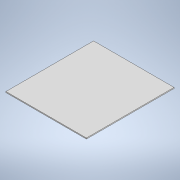
# Autodesk Inventor part: casing lidN
Saved by Autodesk Inventor 2022 (Build 260153000, 153)
## iProperties
Created: 2023-02-15
Part Number: casing lidN
Material: Generic
Document SubType Name: Modeling
Designer: biom
Density: 1 g/cm^3
Appearance: Default
Author: biom
Autodesk Inventor part; units mm, degrees
ref_plane "YZ Plane" through (0, 0, 0) normal (1, 0, 0) x (0, 1, 0)
ref_plane "XZ Plane" through (0, 0, 0) normal (0, 1, 0) x (-1, 0, 0)
ref_plane "XY Plane" through (0, 0, 0) normal (0, 0, 1) x (1, 0, 0)
sketch "Sketch1" plane through (0, 0, 0) normal (0, 1, 0) x (-1, 0, 0)
  line L0 (0, 0) -> (101.5, 0)
  line L1 (101.5, 0) -> (101.5, -110.5)
  line L2 (101.5, -110.5) -> (0, -110.5)
  line L3 (0, -110.5) -> (0, 0)
  dimension "d0" = 101.5
  dimension "d1" = 110.5
  constraints: 8 end point, 2 parallel, 1 horizontal, 1 perpendicular
  measures "d0" distance of L1.end L2.end
  measures "d1" distance of L0.end L1.end
extrude "Extrusion1" add sketch "Sketch1" along normal blind 1.25
body "Solid1"
